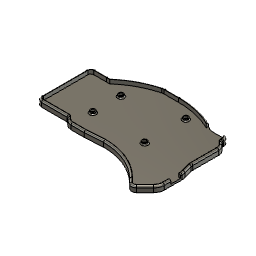
case (Autodesk Fusion 360 design; units mm, degrees)
Autodesk Fusion 360 part; units mm, degrees
note: some values were not read from the file. Set by a fixed rule: which sketch regions a step uses; the direction of a hole.
sketch "outline" plane through (0, 0, 0) normal (0, 1, 0) x (1, 0, 0)
  circle A0 centre (137.6564, -22.162001) radius 0.4064
  circle A1 centre (46.999997, -31.010001) radius 1.1
  circle A2 centre (100.999999, -60.510002) radius 1.1
  circle A3 centre (100.999999, -18.010001) radius 1.1
  circle A4 centre (46.999997, -60.010002) radius 1.1
  circle A5 centre (144.98, -77.620003) radius 0.6
  circle A6 centre (144.98, -79.370003) radius 0.6
  circle A7 centre (121.109999, -23.432001) radius 0.4064
  line L0 (81.999998, -7.50976) -> (67.009997, -7.51)
  arc A8 (67.009997, -7.51) -> (65.098693, -7.769067) centre (67.009998, -14.690002) ccw
  line L1 (26.499996, -26.510001) -> (13.499995, -26.510001)
  spline S0 degree 3 poles (13.499995, -26.510001) (12.395426, -26.510001) (11.499995, -27.405431) (11.499995, -28.510001) knots 11 11 11 11 12 12 12 12
  line L2 (11.499995, -28.510001) -> (11.499995, -74.510003)
  spline S1 degree 3 poles (11.499995, -74.510003) (11.499995, -75.614571) (12.395425, -76.510003) (13.499995, -76.510003) knots 14 14 14 14 15 15 15 15
  line L3 (13.499995, -76.510003) -> (26.499996, -76.510003)
  line L4 (31.499996, -76.510003) -> (39.859996, -76.510003)
  spline S2 degree 3 poles (39.859996, -76.510003) (41.186076, -76.510003) (42.457848, -77.036787) (43.395532, -77.974467) knots 26 26 26 26 27 27 27 27
  line L5 (43.395532, -77.974467) -> (45.464464, -80.045539)
  spline S3 degree 3 poles (45.464464, -80.045539) (46.402144, -80.983219) (47.673917, -81.510003) (48.999997, -81.510003) knots 28 28 28 28 29 29 29 29
  line L6 (48.999997, -81.510003) -> (62.529997, -81.510003)
  line L7 (62.529997, -81.510003) -> (81.149998, -80.218123)
  spline S4 degree 3 poles (81.149998, -80.218123) (99.287647, -80.218123) (116.681383, -87.428116) (129.5, -100.260004) knots 31 31 31 31 32 32 32 32
  line L8 (129.5, -100.260004) -> (134.074672, -104.81114)
  spline S5 degree 3 poles (134.074672, -104.81114) (134.870096, -105.586812) (136.143568, -105.57134) (136.919904, -104.77658) knots 33 33 33 33 34 34 34 34
  line L9 (136.919904, -104.77658) -> (145.670816, -96.022788)
  spline S6 degree 3 poles (145.670816, -96.022788) (147.190065, -94.509372) (148.045873, -92.45442) (148.050001, -90.310004) knots 35 35 35 35 36 36 36 36
  line L10 (148.050001, -90.310004) -> (148.046401, -71.986243)
  arc A9 (148.046401, -71.986243) -> (147.690001, -69.380003) centre (138.046449, -72.026235) ccw
  line L11 (147.690001, -69.380003) -> (145.35, -60.626238)
  arc A10 (145.35, -60.626238) -> (144.9936, -58.020002) centre (154.993522, -57.98001) cw
  line L12 (144.9936, -58.020002) -> (144.994464, -31.115535)
  spline S7 degree 3 poles (144.994464, -31.115535) (144.994464, -29.789453) (144.46768, -28.517683) (143.53, -27.580001) knots 41 41 41 41 42 42 42 42
  line L13 (143.53, -27.580001) -> (140.964464, -25.015535)
  spline S8 degree 3 poles (140.964464, -25.015535) (140.026784, -24.077853) (139.5, -22.806083) (139.5, -21.480001) knots 43 43 43 43 44 44 44 44
  line L14 (139.5, -21.480001) -> (139.5, -20.320001)
  spline S9 degree 3 poles (139.5, -20.320001) (139.5, -19.215431) (138.604576, -18.320001) (137.5, -18.320001) knots 45 45 45 45 46 46 46 46
  line L15 (137.5, -18.320001) -> (125.99, -18.322097)
  arc A11 (125.99, -18.322097) -> (120.139999, -16.700001) centre (125.968068, -7.041292) cw
  spline S10 degree 3 poles (120.139999, -16.700001) (108.333783, -10.659615) (95.26171, -7.50976) (81.999998, -7.50976) knots 49 49 49 49 50 50 50 50
  line L16 (26.499996, -26.510001) -> (30.222016, -26.510001)
  line L17 (26.499996, -76.510003) -> (31.499996, -76.510003)
  spline S11 degree 3 poles (65.098693, -7.769067) (52.164078, -11.198456) (40.217888, -17.618602) (30.222016, -26.510001) knots 2 2 2 2 2.99104371 2.99104371 2.99104371 2.99104371
  circle A12 centre (46.999997, -31.010001) radius 2.5
  circle A13 centre (46.999997, -60.010002) radius 2.5
  circle A14 centre (100.999999, -60.510002) radius 2.5
  circle A15 centre (100.999999, -18.010001) radius 2.5
  line L18 (139.101517, -20.819072) -> (119.101517, -20.819072)
  line L19 (119.101517, -20.819072) -> (119.101517, -8.987749)
  line L20 (119.101517, -8.987749) -> (139.101517, -8.987749)
  line L21 (139.101517, -8.987749) -> (139.101517, -20.819072)
  line L22 (153.296785, -83.495003) -> (138.046449, -83.495003)
  line L23 (138.046449, -83.495003) -> (138.046449, -73.495003)
  line L24 (138.046449, -73.495003) -> (153.296785, -73.495003)
  line L25 (153.296785, -73.495003) -> (153.296785, -83.495003)
  line L26 (144.98, -79.370003) -> (144.98, -83.495003)
  line L27 (144.98, -77.620003) -> (144.98, -73.495003)
  spline S12 degree 3 poles (133.372933, -105.523592) (133.374126, -105.524755) (133.375318, -105.525918) (133.37651, -105.52708) (134.422921, -106.547507) (136.044054, -106.655076) (137.208606, -105.838145) (137.357966, -105.73337) (137.499588, -105.613665) (137.630811, -105.479886) knots 32.99850101 32.99850101 32.99850101 32.99850101 33 33 33 33.88518752 33.88518752 33.88518752 33.9987175 33.9987175 33.9987175 33.9987175
  line L28 (137.630811, -105.479886) -> (146.376562, -96.731253)
  spline S13 degree 3 poles (146.376562, -96.731253) (148.083437, -95.03093) (149.045361, -92.721171) (149.049999, -90.311929) knots 35 35 35 35 36 36 36 36
  line L29 (149.049999, -90.311929) -> (149.0464, -71.98419)
  arc A16 (149.0464, -71.98419) -> (148.655247, -69.118642) centre (138.046449, -72.026235) ccw
  line L30 (148.655247, -69.118642) -> (146.315204, -60.364717)
  arc A17 (145.993601, -58.017966) -> (146.315204, -60.364717) centre (154.993522, -57.98001) ccw
  line L31 (145.993601, -58.017966) -> (145.994464, -31.115535)
  spline S14 degree 3 poles (145.994464, -31.115535) (145.994464, -29.524621) (145.362052, -27.997842) (144.237108, -26.872895) knots 41 41 41 41 42 42 42 42
  line L32 (144.237108, -26.872895) -> (141.671572, -24.308429)
  spline S15 degree 3 poles (141.671572, -24.308429) (140.921156, -23.558012) (140.5, -22.541251) (140.5, -21.480001) knots 43 43 43 43 44 44 44 44
  line L33 (140.5, -21.480001) -> (140.5, -20.320001)
  spline S16 degree 3 poles (140.5, -20.320001) (140.5, -18.865042) (139.450251, -17.634902) (138.058968, -17.372165) (137.877238, -17.337846) (137.690049, -17.320001) (137.5, -17.320001) knots 45 45 45 45 45.88446993 45.88446993 45.88446993 46 46 46 46
  line L34 (137.5, -17.320001) -> (125.988916, -17.322097)
  arc A18 (120.627375, -15.826073) -> (125.988916, -17.322097) centre (125.968068, -7.041292) ccw
  spline S17 degree 3 poles (120.627375, -15.826073) (120.616742, -15.820633) (120.606108, -15.815193) (120.595475, -15.809752) (108.648294, -9.697246) (95.420054, -6.50976) (81.999998, -6.50976) knots 48.99909934 48.99909934 48.99909934 48.99909934 49 49 49 50 50 50 50
  line L35 (81.999998, -6.50976) -> (67.009989, -6.51)
  arc A19 (67.009989, -6.51) -> (64.837596, -6.803742) centre (67.009998, -14.690002) ccw
  spline S18 degree 3 poles (64.837596, -6.803742) (51.876334, -10.240996) (39.896172, -16.646681) (29.842885, -25.510001) knots 2.00012167 2.00012167 2.00012167 2.00012167 2.98173489 2.98173489 2.98173489 2.98173489
  line L36 (26.499996, -25.510001) -> (29.842885, -25.510001)
  line L37 (26.499996, -25.510001) -> (13.499995, -25.510001)
  spline S19 degree 3 poles (13.499995, -25.510001) (12.044994, -25.510001) (10.81483, -26.559813) (10.552138, -27.951149) (10.517833, -28.132843) (10.499995, -28.319993) (10.499995, -28.510001) knots 11 11 11 11 11.88449419 11.88449419 11.88449419 12 12 12 12
  line L38 (10.499995, -28.510001) -> (10.499995, -74.510003)
  spline S20 degree 3 poles (10.499995, -74.510003) (10.499995, -75.965009) (11.549814, -77.195177) (12.941159, -77.457863) (13.122848, -77.492166) (13.309993, -77.510003) (13.499995, -77.510003) knots 14 14 14 14 14.88449765 14.88449765 14.88449765 15 15 15 15
  line L39 (13.499995, -77.510003) -> (26.499996, -77.510003)
  line L40 (26.499996, -77.510003) -> (31.499996, -77.510003)
  line L41 (31.499996, -77.510003) -> (39.859996, -77.510003)
  spline S21 degree 3 poles (39.859996, -77.510003) (40.921244, -77.510003) (41.938008, -77.931159) (42.688427, -78.681575) knots 26 26 26 26 27 27 27 27
  line L42 (42.688427, -78.681575) -> (44.757358, -80.752646)
  spline S22 degree 3 poles (44.757358, -80.752646) (45.882303, -81.877592) (47.409084, -82.510003) (48.999997, -82.510003) knots 28 28 28 28 29 29 29 29
  line L43 (48.999997, -82.510003) -> (62.564646, -82.510003)
  line L44 (62.564646, -82.510003) -> (81.18452, -81.218132)
  spline S23 degree 3 poles (81.18452, -81.218132) (99.044704, -81.227274) (116.169337, -88.330485) (128.792527, -100.966745) (128.792892, -100.96711) (128.793257, -100.967475) (128.793621, -100.96784) knots 31.00064386 31.00064386 31.00064386 31.00064386 32 32 32 32.00002845 32.00002845 32.00002845 32.00002845
  line L45 (128.793621, -100.96784) -> (133.372933, -105.523592)
  spline S24 degree 3 poles (131.969456, -106.948496) (131.973033, -106.951984) (131.97661, -106.955472) (131.980187, -106.95896) (133.100149, -108.051111) (134.641845, -108.524976) (136.096998, -108.34488) (137.176107, -108.211324) (138.237551, -107.713929) (139.051122, -106.888) knots 32.99550302 32.99550302 32.99550302 32.99550302 33 33 33 33.57270759 33.57270759 33.57270759 33.99741485 33.99741485 33.99741485 33.99741485
  line L46 (139.051122, -106.888) -> (147.788053, -98.148184)
  spline S25 degree 3 poles (147.788053, -98.148184) (149.870182, -96.074047) (151.044338, -93.254674) (151.049995, -90.315779) (151.049997, -90.314718) (151.049999, -90.313657) (151.050001, -90.312596) knots 35 35 35 35 36 36 36 36.00049465 36.00049465 36.00049465 36.00049465
  line L47 (151.050001, -90.312596) -> (151.046399, -71.980323)
  arc A20 (151.046399, -71.980323) -> (150.585847, -68.596319) centre (138.046449, -72.026235) ccw
  line L48 (150.585847, -68.596319) -> (148.245451, -59.841075)
  arc A21 (147.993601, -58.013514) -> (148.245451, -59.841075) centre (154.993522, -57.98001) ccw
  line L49 (147.993601, -58.013514) -> (147.994464, -31.115535)
  spline S26 degree 3 poles (147.994464, -31.115535) (147.994464, -28.994956) (147.150796, -26.958159) (145.651323, -25.458683) knots 41 41 41 41 42 42 42 42
  line L50 (145.651323, -25.458683) -> (143.085787, -22.894217)
  spline S27 degree 3 poles (143.085787, -22.894217) (142.7099, -22.518329) (142.5, -22.011586) (142.5, -21.480001) knots 43 43 43 43 44 44 44 44
  line L51 (142.5, -21.480001) -> (142.5, -20.320001)
  spline S28 degree 3 poles (142.5, -20.320001) (142.5, -18.760583) (141.76554, -17.330282) (140.624763, -16.416591) (139.77145, -15.733141) (138.666464, -15.320001) (137.5, -15.320001) knots 45 45 45 45 45.57207916 45.57207916 45.57207916 46 46 46 46
  line L52 (137.5, -15.320001) -> (125.986606, -15.322097)
  arc A22 (121.607178, -14.080803) -> (125.986606, -15.322097) centre (125.968068, -7.041292) ccw
  spline S29 degree 3 poles (121.607178, -14.080803) (121.573594, -14.063621) (121.54001, -14.046438) (121.506426, -14.029256) (109.277315, -7.772506) (95.73674, -4.50976) (81.999998, -4.50976) (81.99999, -4.50976) (81.999982, -4.50976) (81.999974, -4.50976) knots 48.9971554 48.9971554 48.9971554 48.9971554 49 49 49 50 50 50 50.0000006 50.0000006 50.0000006 50.0000006
  line L53 (81.999974, -4.50976) -> (67.009973, -4.51)
  arc A23 (67.009973, -4.51) -> (64.316128, -4.8729) centre (67.009998, -14.690002) ccw
  spline S30 degree 3 poles (64.316128, -4.8729) (51.303176, -8.325296) (39.256925, -14.702327) (29.09207, -23.510001) knots 2.00033881 2.00033881 2.00033881 2.00033881 2.96360874 2.96360874 2.96360874 2.96360874
  line L54 (26.499996, -23.510001) -> (29.09207, -23.510001)
  line L55 (26.499996, -23.510001) -> (13.499995, -23.510001)
  spline S31 degree 3 poles (13.499995, -23.510001) (11.940606, -23.510001) (10.510336, -24.244434) (9.596647, -25.385164) (8.913162, -26.238487) (8.499995, -27.343501) (8.499995, -28.510001) knots 11 11 11 11 11.57206623 11.57206623 11.57206623 12 12 12 12
  line L56 (8.499995, -28.510001) -> (8.499995, -74.510003)
  spline S32 degree 3 poles (8.499995, -74.510003) (8.499995, -76.069395) (9.23443, -77.499665) (10.375163, -78.413355) (11.228485, -79.096837) (12.333496, -79.510003) (13.499995, -79.510003) knots 14 14 14 14 14.57206715 14.57206715 14.57206715 15 15 15 15
  line L57 (13.499995, -79.510003) -> (26.499996, -79.510003)
  line L58 (26.499996, -79.510003) -> (31.499996, -79.510003)
  line L59 (31.499996, -79.510003) -> (39.859996, -79.510003)
  spline S33 degree 3 poles (39.859996, -79.510003) (40.391578, -79.510003) (40.898327, -79.719904) (41.274217, -80.095792) knots 26 26 26 26 27 27 27 27
  line L60 (41.274217, -80.095792) -> (43.343144, -82.16686)
  spline S34 degree 3 poles (43.343144, -82.16686) (44.842621, -83.666337) (46.879418, -84.510003) (48.999997, -84.510003) knots 28 28 28 28 29 29 29 29
  line L61 (48.999997, -84.510003) -> (62.633944, -84.510003)
  line L62 (62.633944, -84.510003) -> (81.252781, -83.218204)
  spline S35 degree 3 poles (81.252781, -83.218204) (98.558304, -83.245385) (115.145062, -90.135041) (127.377582, -102.380226) (127.378676, -102.381322) (127.379771, -102.382417) (127.380865, -102.383512) knots 31.00197571 31.00197571 31.00197571 31.00197571 32 32 32 32.00008536 32.00008536 32.00008536 32.00008536
  line L63 (127.380865, -102.383512) -> (131.969456, -106.948496)
  dimension "d46" = 5
  dimension "d47" = 5
  dimension "d48" = 5
  dimension "d49" = 5
  dimension "d50" = 20
  dimension "d51" = 10
  dimension "d54" = 1
  dimension "d55" = 3
  constraint parallel L1 L16
  constraint concentric A1 A12
  constraint concentric A4 A13
  constraint concentric A2 A14
  constraint concentric A3 A15
  constraint horizontal L18
  constraint vertical L19
  constraint horizontal L20
  constraint vertical L21
  constraint horizontal L22
  constraint vertical L23
  constraint horizontal L24
  constraint vertical L25
  constraint perpendicular L22 L26
  constraint perpendicular L24 L27
  constraint equal L26 L27
  measures "d46" diameter of A12
  measures "d47" diameter of A13
  measures "d48" diameter of A14
  measures "d49" diameter of A15
extrude "Extrude12" add sketch "outline" along normal blind 4 contours A1 | A2 | A3 | A4 | A12 | A13 | A14 | A15 picked at (47.660577, -31.18888) picked at (100.751364, -61.063842) picked at (101.183332, -17.476304) picked at (46.486308, -59.755353) picked at (49.019927, -31.188852) picked at (49.019927, -60.188853) picked at (99.397636, -61.752797) picked at (103.019929, -18.188851) makes body 1 at (49.496889, 2.666667, 60.134617) makes body 2 at (49.496889, 2.666667, 31.134616) makes body 3 at (99.007167, 2.666667, 62.019513) makes body 4 at (103.496891, 2.666667, 18.134615)
hole "Hole2" at (46.999997, 0, 31.010001) at (100.999999, 0, 18.010001) at (100.999999, 0, 60.510002) at (46.999997, 0, 60.010002) direction (0, 1, 0) diameter 3.3 end through all bodies 2 1 3 4
extrude "Extrude8" add sketch "outline" along normal blind 6 separate body contours L19 L22 S12 L28 S13 L29 S17 L35 A19 S18 L36 L37 S19 L38 S20 L39 L40 L41 S21 L42 S22 L43 L44 S23 L45 S24 L46 S25 L47 S29 L53 A23 S30 L54 L55 S31 L56 S32 L57 L58 L59 S33 L60 S34 L61 L62 S35 L63 | L19 L21 S16 L34 A18 S17 S28 L52 A22 S29 | L21 L24 L29 A16 L30 A17 L31 S14 L32 S15 L33 S16 L47 A20 L48 A21 L49 S26 L50 S27 L51 S28 | L22 L24 L29 L47 picked at (104.300152, -8.960954) picked at (129.825174, -15.988065) picked at (146.660555, -49.049005) picked at (150.38134, -80.16167) makes body 5
extrude "Extrude11" cut sketch "outline" along normal blind 10 from surface at 2 contours S9 L15 A11 S10 L19 L21 S16 L34 A18 S17 | S9 L15 A11 S10 L18 L19 L21 | L19 L21 S16 L34 A18 S17 S28 L52 A22 S29 | L19 L20 L21 S28 L52 A22 S29 | L10 L22 L24 L29 | L10 L22 L23 L24 | L22 L24 L29 L47 | L22 L24 L25 L47 picked at (129.826305, -17.654731) picked at (128.064344, -19.986747) picked at (129.825174, -15.988065) picked at (128.063213, -11.099199) picked at (148.380685, -76.828336) picked at (140.161476, -78.242355) picked at (150.38134, -80.16167) picked at (151.797381, -76.828336) bodies 5
extrude "Extrude9" add sketch "outline" along normal blind 2 contours A0 | A1 | A2 | A3 | A4 | A5 | A6 | A7 | L0 A8 L1 S0 L2 S1 L3 L4 S2 L5 S3 L6 L7 S4 L8 S5 L9 S6 L10 A9 L11 A10 L12 S7 L13 S8 L14 S9 S10 L16 L17 S11 L18 L19 L21 L22 L23 L24 | L0 A8 L1 S0 L2 S1 L3 L4 S2 L5 S3 L6 L7 S4 L8 S5 L9 S6 L10 S10 L16 L17 S11 L19 L22 S12 L28 S13 L29 S17 L35 A19 S18 L36 L37 S19 L38 S20 L39 L40 L41 S21 L42 S22 L43 L44 S23 L45 | S9 L15 A11 S10 L19 L21 S16 L34 A18 S17 | S9 L15 A11 S10 L18 L19 L21 | L19 L22 S12 L28 S13 L29 S17 L35 A19 S18 L36 L37 S19 L38 S20 L39 L40 L41 S21 L42 S22 L43 L44 S23 L45 S24 L46 S25 L47 S29 L53 A23 S30 L54 L55 S31 L56 S32 L57 L58 L59 S33 L60 S34 L61 L62 S35 L63 | L19 L21 S16 L34 A18 S17 S28 L52 A22 S29 | L10 A9 L11 A10 L12 S7 L13 S8 L14 S9 L21 L24 L29 A16 L30 A17 L31 S14 L32 S15 L33 S16 | L21 L24 L29 A16 L30 A17 L31 S14 L32 S15 L33 S16 L47 A20 L48 A21 L49 S26 L50 S27 L51 S28 | L10 L22 L24 L29 | L10 L22 L23 L24 | L22 L24 L29 L47 | A12 | A13 | A14 | A15 picked at (137.724133, -22.004303) picked at (47.660577, -31.18888) picked at (100.751364, -61.063842) picked at (101.183332, -17.476304) picked at (46.486308, -59.755353) picked at (144.640867, -77.761158) picked at (144.640867, -79.228848) picked at (121.239448, -23.47193) picked at (82.574556, -36.755631) picked at (115.54606, -14.344525) picked at (129.826305, -17.654731) picked at (128.064344, -19.986747) picked at (104.300152, -8.960954) picked at (129.825174, -15.988065) picked at (145.327222, -49.051168) picked at (146.660555, -49.049005) picked at (148.380685, -76.828336) picked at (140.161476, -78.242355) picked at (150.38134, -80.16167) picked at (49.019927, -31.188852) picked at (49.019927, -60.188853) picked at (99.397636, -61.752797) picked at (103.019929, -18.188851) bodies 1 2 3 4 5
fillet "Fillet3" radius 1.8 31 edges at (106.219569, 6, 88.218299) (71.943363, 6, 83.864104) (27.796033, 6, 23.510001) (19.999995, 6, 23.510001) (9.965773, 6, 24.974052) (8.499995, 6, 51.510002) (9.964046, 6, 78.044224) (26.679996, 6, 79.510003) (40.625491, 6, 79.66194) (42.30868, 6, 81.131326) (45.938658, 6, 83.900735) (55.81697, 6, 84.510003) (45.636063, 6, 12.183221) (101.021088, 6, 6.621106) (74.504973, 6, 4.50988) (65.650884, 6, 4.601135) (147.994033, 6, 44.564525) (147.385196, 6, 28.054196) (144.368555, 6, 24.17645) (142.651936, 6, 22.245495) (142.5, 6, 20.900001) (141.542764, 6, 17.381504) (149.415649, 6, 64.218697) (148.059056, 6, 58.935628) (150.927732, 6, 70.273131) (151.046548, 6, 72.737663) (151.049331, 6, 86.9038) (150.198524, 6, 94.55429) (143.419588, 6, 102.518092) (135.512391, 6, 108.382121) (129.67516, 6, 104.666004) on bodies 1 5
chamfer "Chamfer3" distance 1 angle 45 4 edges at (44.669178, 2, 31.91404) (44.669178, 2, 60.914041) (98.66918, 2, 61.414041) (98.66918, 2, 18.914039) on bodies 1
